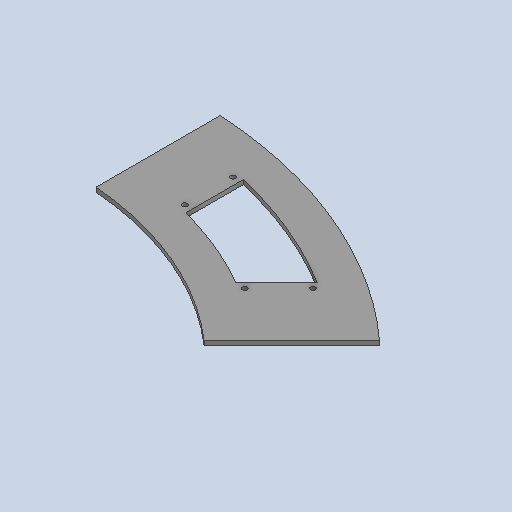
# Autodesk Inventor part: Battery Module Third Iteration
Saved by Autodesk Inventor 2023 (Build 270158000, 158)
## iProperties
Created: 2023-03-05
Part Number: Battery Module Third Iteration
Material: PLA Plastic
Document SubType Name: Modeling
Designer: mihal
Density: 1.25002 g/cm^3
Appearance: Generic
Mass: 44.3782 g
Surface Area: 260.707 cm^2
Volume: 35.5018 cm^3
Author: mihal
Autodesk Inventor part; units mm, degrees
ref_plane "YZ Plane" through (0, 0, 0) normal (1, 0, 0) x (0, 1, 0)
ref_plane "XZ Plane" through (0, 0, 0) normal (0, 1, 0) x (-1, 0, 0)
ref_plane "XY Plane" through (0, 0, 0) normal (0, 0, 1) x (1, 0, 0)
sketch "Sketch1" plane through (0, 0, 0) normal (0, 1, 0) x (-1, 0, 0)
  circle A0 centre (0, 0) radius 215
  circle A1 centre (0, 0) radius 315
  line L0 (0, 0) -> (0, -315)
  line L1 (0, 0) -> (-222.7386, -222.7386)
  line L2 (-141.0509, -162.2641) -> (-211.8794, -233.0926)
  line L3 (-15, -214.4761) -> (-15, -314.6427)
  circle A2 centre (0, 0) radius 222.5
  circle A3 centre (0, 0) radius 307.5
  line L4 (-18, -214.2452) -> (-18, -314.4853)
  point P0 (-152.028, -152.028)
  point P1 (0, -215)
  point P2 (0, -312.5)
  point P3 (0, -217.5)
  point P4 (-153.7957, -153.7957)
  point P5 (-220.9709, -220.9709)
  point P6 (-210.1096, -231.3228)
  point P7 (-15, -312.1398)
  point P8 (-15, -216.9821)
  point P9 (-142.8229, -164.0361)
  point P10 (-206.5699, -227.7831)
  point P11 (-15, -307.1339)
  point P12 (-15, -221.9938)
  point P13 (-146.3667, -167.5799)
  point P14 (-18, -306.9727)
  point P15 (-18, -221.7707)
  dimension "d2" = 430
  dimension "d3" = 630
  dimension "d4" = 45
  dimension "d5" = 15
  dimension "d6" = 15
  dimension "d11" = 7.5
  dimension "d12" = 7.5
  dimension "d13" = 3
  constraints: 10 end point, 8 point on circle, 4 centre point, 4 coincident, 3 parallel, 2 vertical
  measures "d2" diameter of A0
  measures "d3" diameter of A1
  measures "d4" angle of L1 L0
  measures "d5" distance between parallel lines of L2 L1
  measures "d6" distance between parallel lines of L3 L0
  measures "d11" radial gap between concentric circles of A0 A2
  measures "d12" radial gap between concentric circles of A3 A1
  measures "d13" distance between parallel lines of L3 L4
extrude "Extrusion1" add sketch "Sketch1" along normal blind 3 contours A2 L4 A3 L2
sketch "Sketch5" plane through (0, 3, 0) normal (0, 1, 0) x (1, 0, 0)
  arc A0 (146.3667, 167.5799) -> (18, 221.7707) centre (0, 0) ccw projected
  line L0 (146.3667, 167.5799) -> (206.5699, 227.7831) projected
  arc A1 (206.5699, 227.7831) -> (18, 306.9727) centre (0, 0) ccw projected
  line L1 (18, 306.9727) -> (18, 221.7707) projected
  circle A2 centre (0, 0) radius 297.5
  circle A3 centre (0, 0) radius 232.5
  line L2 (28, 296.1794) -> (28, 230.8078)
  line L3 (145.7715, 181.1268) -> (191.9425, 227.2979)
  line L4 (18, 306.9727) -> (18, 221.7707) projected
  line L5 (18, 296.955) -> (18, 231.8022)
  line L6 (146.3667, 167.5799) -> (206.5699, 227.7831) projected
  line L7 (199.4901, 220.7033) -> (153.4532, 174.6664)
  dimension "d43" = 10
  dimension "d44" = 10
  dimension "d45" = 10
  dimension "d46" = 10
  constraints: 8 end point, 8 point on circle, 4 point on line, 2 centre point, 2 coincident, 1 parallel, 1 vertical
  measures "d43" radial gap between concentric circles of A0 A3
  measures "d44" radial gap between concentric circles of A1 A2
  measures "d45" distance between parallel lines of L2 L5
  measures "d46" distance between parallel lines of L0 L3
sketch "Sketch6" plane through (0, 3, 0) normal (0, 1, 0) x (1, 0, 0)
  arc A0 (146.3667, 167.5799) -> (18, 221.7707) centre (0, 0) ccw projected
  line L0 (146.3667, 167.5799) -> (206.5699, 227.7831) projected
  arc A1 (206.5699, 227.7831) -> (18, 306.9727) centre (0, 0) ccw projected
  line L1 (18, 306.9727) -> (18, 221.7707) projected
  circle A2 centre (0, 0) radius 222.5
  circle A3 centre (0, 0) radius 309.5
  circle A4 centre (0, 0) radius 240
  circle A5 centre (0, 0) radius 290
  line L2 (18, 306.9727) -> (18, 221.7707) projected
  line L3 (18, 239.324) -> (18, 289.4408)
  line L4 (146.3667, 167.5799) -> (206.5699, 227.7831) projected
  line L5 (158.7672, 179.9804) -> (194.1799, 215.3931)
  line L6 (50, 234.7339) -> (50, 285.6571)
  line L7 (130.6266, 201.3373) -> (166.6348, 237.3454)
  line L8 (55, 233.6129) -> (55, 284.7367)
  line L9 (126.2984, 204.0802) -> (162.4484, 240.2301)
  circle A6 centre (0, 0) radius 245
  circle A7 centre (0, 0) radius 285
  line L10 (55, 274.8261) -> (59, 274.8261) construction
  line L11 (59, 274.8261) -> (59, 278.8261) construction
  line L12 (55, 241.7898) -> (59, 241.7898) construction
  line L13 (59, 241.7898) -> (59, 237.7898) construction
  line L14 (132.0804, 209.8621) -> (129.2519, 212.6905) construction
  line L15 (129.2519, 212.6905) -> (126.4235, 209.8621) construction
  line L16 (155.4405, 233.2223) -> (152.6121, 236.0507) construction
  line L17 (152.6121, 236.0507) -> (155.4405, 238.8791) construction
  circle A8 centre (152.6121, 236.0507) radius 1.75
  circle A9 centre (129.2519, 212.6905) radius 1.75
  circle A10 centre (59, 274.8261) radius 1.75
  circle A11 centre (59, 241.7898) radius 1.75
  line L18 (15, 221.9938) -> (15, 309.1363)
  line L19 (0, 449.6314) -> (0, -436.0219) projected
  point P0 (176.4736, 197.6868)
  dimension "d47" = 445
  dimension "d48" = 619
  dimension "d49" = 480
  dimension "d50" = 580
  dimension "d53" = 5
  dimension "d54" = 5
  dimension "d55" = 5
  dimension "d56" = 5
  dimension "d57" = 4
  dimension "d58" = 4
  dimension "d59" = 4
  dimension "d60" = 4
  dimension "d61" = 4
  dimension "d63" = 4
  dimension "d67" = 90
  dimension "d68" = 4
  dimension "d69" = 4
  dimension "d70" = 3.5
  dimension "d71" = 3.5
  dimension "d72" = 3.5
  dimension "d73" = 3.5
  dimension "d76" = 35
  dimension "d77" = 15
  dimension "d78" = 35
  constraints: 30 end point, 16 point on circle, 10 coincident, 8 centre point, 8 point on line, 5 perpendicular, 4 parallel, 2 horizontal, 1 midpoint, 1 vertical, 7 other
  measures "d49" diameter of A4
  measures "d50" diameter of A5
  measures "d53" distance between parallel lines of L6 L8
  measures "d54" distance between parallel lines of L9 L7
  measures "d55" radial gap between concentric circles of A5 A7
  measures "d56" radial gap between concentric circles of A4 A6
  measures "d57" distance of L10.start L10.end
  measures "d58" distance of L10.end L11.end
  measures "d59" distance of L12.end L13.end
  measures "d60" distance of L12.start L12.end
  measures "d61" distance of L14.start L14.end
  measures "d63" distance of L14.end L15.end
  measures "d67" angle of L9 L16
  measures "d68" distance of L16.start L16.end
  measures "d69" distance of L16.end L17.end
  measures "d70" diameter of A8
  measures "d71" diameter of A9
  measures "d72" diameter of A10
  measures "d73" diameter of A11
  measures "d76" distance between parallel lines of L0 L7
  measures "d77" distance between parallel lines of L19 L18
  measures "d78" distance between parallel lines of L18 L6
extrude "Extrusion4" cut sketch "Sketch6" against normal up to next contours A8 | A9 | A10 | A11
sketch "Sketch8" plane through (0, 3, 0) normal (0, 1, 0) x (1, 0, 0)
  circle A0 centre (129.2519, 212.6905) radius 1.75 projected
  circle A1 centre (59, 274.8261) radius 1.75 projected
  circle A2 centre (152.6121, 236.0507) radius 1.75 projected
  circle A3 centre (59, 241.7898) radius 1.75 projected
  arc A4 (146.3667, 167.5799) -> (18, 221.7707) centre (0, 0) ccw projected
  line L0 (146.3667, 167.5799) -> (206.5699, 227.7831) projected
  arc A5 (206.5699, 227.7831) -> (18, 306.9727) centre (0, 0) ccw projected
  line L1 (18, 306.9727) -> (18, 221.7707) projected
  circle A6 centre (129.2519, 212.6905) radius 1.75 projected
  circle A7 centre (59, 241.7898) radius 1.75 projected
  circle A8 centre (152.6121, 236.0507) radius 1.75 projected
  circle A9 centre (0, 0) radius 248.8841 construction
  circle A10 centre (59, 274.8261) radius 1.75 projected
  circle A11 centre (0, 0) radius 281.0879 construction
  circle A12 centre (0, 0) radius 245.8841
  circle A13 centre (0, 0) radius 284.0879
  line L2 (59, 241.7898) -> (59, 274.8261) construction
  line L3 (129.2519, 212.6905) -> (152.6121, 236.0507) construction
  line L4 (122.6187, 213.1283) -> (150.4617, 240.9714)
  line L5 (64, 237.409) -> (64, 276.785)
  dimension "d96" = 3
  dimension "d97" = 3
  dimension "d98" = 5
  dimension "d100" = 5
  constraints: 8 end point, 4 coincident, 4 point on circle, 2 centre point, 2 parallel, 1 vertical, 6 other
  measures "d98" distance between parallel lines of L3 L4
  measures "d100" distance between parallel lines of L5 L2
extrude "Extrusion5" cut sketch "Sketch8" against normal up to next contours A0 | A1 | A2 | A3 | A12 L5 A13 L4
body "Solid1"
